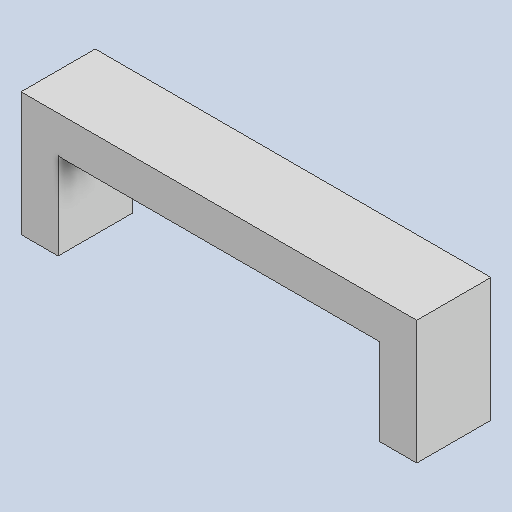
# Autodesk Inventor part: thing
Saved by Autodesk Inventor 2025.2 (Build 292293000, 293)
## iProperties
Created: 2025-03-30
Part Number: thing
Material: Generic
Document SubType Name: Modeling
Designer: mirewn
Density: 1 g/cm^3
Appearance: Default
Author: mirewn
Autodesk Inventor part; units mm, degrees
ref_plane "YZ Plane" through (0, 0, 0) normal (1, 0, 0) x (0, 1, 0)
ref_plane "XZ Plane" through (0, 0, 0) normal (0, 1, 0) x (-1, 0, 0)
ref_plane "XY Plane" through (0, 0, 0) normal (0, 0, 1) x (1, 0, 0)
sketch "Sketch1" plane through (0, 0, 0) normal (0, 0, 1) x (1, 0, 0)
  line L0 (0, 0) -> (1.5, 0)
  line L1 (1.5, 0) -> (1.5, 3.5)
  line L2 (1.5, 3.5) -> (14.5, 3.5)
  line L3 (14.5, 3.5) -> (14.5, 0)
  line L4 (14.5, 0) -> (16, 0)
  line L5 (16, 0) -> (16, 5)
  line L6 (16, 5) -> (0, 5)
  line L7 (0, 5) -> (0, 0)
  point P0 (15.25, 0)
  dimension "d0" = 1.5
  dimension "d1" = 3.5
  dimension "d2" = 13
  dimension "d3" = 1.5
  dimension "d7" = 1.5
  constraints: 16 end point, 6 perpendicular, 2 horizontal, 1 horizontal alignment, 1 midpoint
  measures "d0" distance of L0.start L0.end
  measures "d1" distance of L0.end L1.end
  measures "d2" distance of L1.end L2.end
  measures "d3" distance of L3.end L4.end
  measures "d7" distance between parallel lines of L6 L2
extrude "Extrusion1" add sketch "Sketch1" along normal blind 3
body "Solid1"
